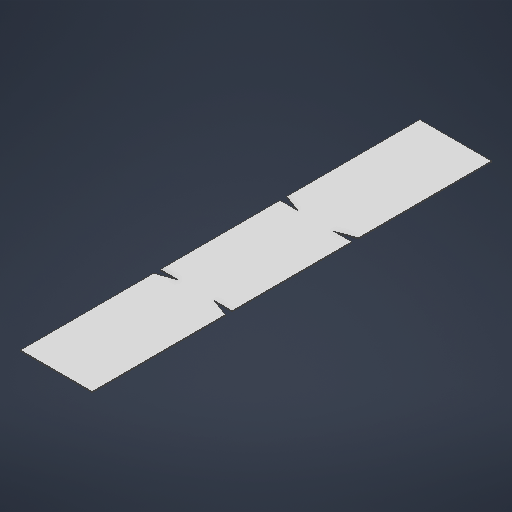
# Autodesk Inventor part: CARDBOARD
Saved by Autodesk Inventor 2025 (Build 290162000, 162)
## iProperties
Created: 2024-05-27
Part Number: CARDBOARD
Material: Generic
Document SubType Name: Modeling
Designer: zulet
Density: 1 g/cm^3
Appearance: Default
Author: zulet
Autodesk Inventor part; units mm, degrees
ref_plane "YZ Plane" through (0, 0, 0) normal (1, 0, 0) x (0, 1, 0)
ref_plane "XZ Plane" through (0, 0, 0) normal (0, 1, 0) x (-1, 0, 0)
ref_plane "XY Plane" through (0, 0, 0) normal (0, 0, 1) x (1, 0, 0)
sketch "Sketch1" plane through (0, 0, 0) normal (0, 1, 0) x (-1, 0, 0)
  line L0 (-90, -500) -> (90, -500)
  line L1 (90, -500) -> (90, 500)
  line L2 (90, 500) -> (-90, 500)
  line L3 (-90, 500) -> (-90, -500)
  line L4 (-90, -500) -> (90, 500) construction
  line L5 (90, -500) -> (-90, 500) construction
  line L6 (-45, -500) -> (45, -500)
  line L7 (45, -500) -> (45, 500) construction
  line L8 (45, 500) -> (-45, 500)
  line L9 (-45, 500) -> (-45, -500) construction
  line L10 (-45, -500) -> (45, 500) construction
  line L11 (45, -500) -> (-45, 500) construction
  line L12 (-90, -150) -> (90, -150) construction
  line L13 (90, -150) -> (90, 150) construction
  line L14 (90, 150) -> (-90, 150) construction
  line L15 (-90, 150) -> (-90, -150) construction
  line L16 (-90, -150) -> (90, 150) construction
  line L17 (90, -150) -> (-90, 150) construction
  line L18 (90, 150) -> (45, 150)
  line L19 (45, 150) -> (90, 166.3787)
  line L20 (0, 0) -> (90, 0) construction
  line L21 (0, 0) -> (0, 150) construction
  line L22 (90, -150) -> (45, -150)
  line L23 (45, -150) -> (90, -166.3787)
  line L24 (-90, 150) -> (-45, 150)
  line L25 (-45, 150) -> (-90, 166.3787)
  line L26 (-90, -150) -> (-45, -150)
  line L27 (-45, -150) -> (-90, -166.3787)
  dimension "d0" = 180
  dimension "d1" = 1000
  dimension "d4" = 90
  dimension "d5" = 300
  dimension "d6" = 20
  constraints: 56 end point, 8 midpoint, 6 parallel, 6 symmetric about line, 5 point on line, 3 horizontal, 3 perpendicular
  measures "d0" distance of L2.end L1.end
  measures "d1" distance of L0.end L1.end
  measures "d4" distance of L8.end L7.end
  measures "d5" distance of L13.end L12.end
  measures "d6" angle of L14 L19
extrude "Extrusion1" add sketch "Sketch1" along normal blind 2 contours L3 L27 L26 L24 L25 L2 L1 L19 L18 L22 L23 L0
body "Solid1"
